Autodesk Fusion 360 part; units mm, degrees
(part 2 of 2)
  arc A318 (288.275, -92.225) -> (288.775, -92.725) centre (288.775, -92.225) ccw
  arc A319 (301.775, -92.725) -> (302.275, -92.225) centre (301.775, -92.225) ccw
  line L320 (5.4062, -97.775) -> (18.4063, -97.775)
  line L321 (5.4062, -111.775) -> (18.4063, -111.775)
  line L322 (4.9062, -98.275) -> (4.9062, -111.275)
  line L323 (18.9062, -98.275) -> (18.9062, -111.275)
  arc A320 (5.4062, -97.775) -> (4.9063, -98.275) centre (5.4062, -98.275) ccw
  arc A321 (18.9062, -98.275) -> (18.4062, -97.775) centre (18.4062, -98.275) ccw
  arc A322 (4.9062, -111.275) -> (5.4062, -111.775) centre (5.4062, -111.275) ccw
  arc A323 (18.4062, -111.775) -> (18.9063, -111.275) centre (18.4062, -111.275) ccw
  line L324 (29.2188, -97.775) -> (42.2188, -97.775)
  line L325 (29.2188, -111.775) -> (42.2188, -111.775)
  line L326 (28.7188, -98.275) -> (28.7188, -111.275)
  line L327 (42.7188, -98.275) -> (42.7188, -111.275)
  arc A324 (29.2188, -97.775) -> (28.7188, -98.275) centre (29.2188, -98.275) ccw
  arc A325 (42.7188, -98.275) -> (42.2188, -97.775) centre (42.2188, -98.275) ccw
  arc A326 (28.7188, -111.275) -> (29.2188, -111.775) centre (29.2188, -111.275) ccw
  arc A327 (42.2188, -111.775) -> (42.7188, -111.275) centre (42.2188, -111.275) ccw
  line L328 (53.0313, -97.775) -> (66.0312, -97.775)
  line L329 (53.0313, -111.775) -> (66.0312, -111.775)
  line L330 (52.5313, -98.275) -> (52.5313, -111.275)
  line L331 (66.5312, -98.275) -> (66.5312, -111.275)
  arc A328 (53.0313, -97.775) -> (52.5313, -98.275) centre (53.0313, -98.275) ccw
  arc A329 (66.5312, -98.275) -> (66.0312, -97.775) centre (66.0312, -98.275) ccw
  arc A330 (52.5313, -111.275) -> (53.0313, -111.775) centre (53.0313, -111.275) ccw
  arc A331 (66.0312, -111.775) -> (66.5312, -111.275) centre (66.0312, -111.275) ccw
  line L332 (124.4688, -97.775) -> (137.4688, -97.775)
  line L333 (124.4688, -111.775) -> (137.4688, -111.775)
  line L334 (123.9688, -98.275) -> (123.9688, -111.275)
  line L335 (137.9688, -98.275) -> (137.9688, -111.275)
  arc A332 (124.4688, -97.775) -> (123.9688, -98.275) centre (124.4688, -98.275) ccw
  arc A333 (137.9688, -98.275) -> (137.4688, -97.775) centre (137.4688, -98.275) ccw
  arc A334 (123.9688, -111.275) -> (124.4688, -111.775) centre (124.4688, -111.275) ccw
  arc A335 (137.4688, -111.775) -> (137.9688, -111.275) centre (137.4688, -111.275) ccw
  line L336 (77.9688, -98.775) -> (83.9688, -98.775)
  line L337 (77.9688, -113.775) -> (83.9688, -113.775)
  line L338 (77.4688, -99.275) -> (77.4688, -113.275)
  line L339 (84.4688, -99.275) -> (84.4688, -113.275)
  arc A336 (77.9688, -98.775) -> (77.4688, -99.275) centre (77.9688, -99.275) ccw
  arc A337 (84.4688, -99.275) -> (83.9688, -98.775) centre (83.9688, -99.275) ccw
  arc A338 (77.4688, -113.275) -> (77.9688, -113.775) centre (77.9688, -113.275) ccw
  arc A339 (83.9688, -113.775) -> (84.4688, -113.275) centre (83.9688, -113.275) ccw
  line L340 (177.9688, -98.775) -> (183.9688, -98.775)
  line L341 (177.9688, -113.775) -> (183.9688, -113.775)
  line L342 (177.4688, -99.275) -> (177.4688, -113.275)
  line L343 (184.4688, -99.275) -> (184.4688, -113.275)
  arc A340 (177.9688, -98.775) -> (177.4688, -99.275) centre (177.9688, -99.275) ccw
  arc A341 (184.4688, -99.275) -> (183.9688, -98.775) centre (183.9688, -99.275) ccw
  arc A342 (177.4688, -113.275) -> (177.9688, -113.775) centre (177.9688, -113.275) ccw
  arc A343 (183.9688, -113.775) -> (184.4688, -113.275) centre (183.9688, -113.275) ccw
  line L344 (193.525, -97.775) -> (206.525, -97.775)
  line L345 (193.525, -111.775) -> (206.525, -111.775)
  line L346 (193.025, -98.275) -> (193.025, -111.275)
  line L347 (207.025, -98.275) -> (207.025, -111.275)
  arc A344 (193.525, -97.775) -> (193.025, -98.275) centre (193.525, -98.275) ccw
  arc A345 (207.025, -98.275) -> (206.525, -97.775) centre (206.525, -98.275) ccw
  arc A346 (193.025, -111.275) -> (193.525, -111.775) centre (193.525, -111.275) ccw
  arc A347 (206.525, -111.775) -> (207.025, -111.275) centre (206.525, -111.275) ccw
  line L348 (212.575, -97.775) -> (225.575, -97.775)
  line L349 (212.575, -111.775) -> (225.575, -111.775)
  line L350 (212.075, -98.275) -> (212.075, -111.275)
  line L351 (226.075, -98.275) -> (226.075, -111.275)
  arc A348 (212.575, -97.775) -> (212.075, -98.275) centre (212.575, -98.275) ccw
  arc A349 (226.075, -98.275) -> (225.575, -97.775) centre (225.575, -98.275) ccw
  arc A350 (212.075, -111.275) -> (212.575, -111.775) centre (212.575, -111.275) ccw
  arc A351 (225.575, -111.775) -> (226.075, -111.275) centre (225.575, -111.275) ccw
  line L352 (231.625, -97.775) -> (244.625, -97.775)
  line L353 (231.625, -111.775) -> (244.625, -111.775)
  line L354 (231.125, -98.275) -> (231.125, -111.275)
  line L355 (245.125, -98.275) -> (245.125, -111.275)
  arc A352 (231.625, -97.775) -> (231.125, -98.275) centre (231.625, -98.275) ccw
  arc A353 (245.125, -98.275) -> (244.625, -97.775) centre (244.625, -98.275) ccw
  arc A354 (231.125, -111.275) -> (231.625, -111.775) centre (231.625, -111.275) ccw
  arc A355 (244.625, -111.775) -> (245.125, -111.275) centre (244.625, -111.275) ccw
  line L356 (250.675, -97.775) -> (263.675, -97.775)
  line L357 (250.675, -111.775) -> (263.675, -111.775)
  line L358 (250.175, -98.275) -> (250.175, -111.275)
  line L359 (264.175, -98.275) -> (264.175, -111.275)
  arc A356 (250.675, -97.775) -> (250.175, -98.275) centre (250.675, -98.275) ccw
  arc A357 (264.175, -98.275) -> (263.675, -97.775) centre (263.675, -98.275) ccw
  arc A358 (250.175, -111.275) -> (250.675, -111.775) centre (250.675, -111.275) ccw
  arc A359 (263.675, -111.775) -> (264.175, -111.275) centre (263.675, -111.275) ccw
  line L360 (269.725, -97.775) -> (282.725, -97.775)
  line L361 (269.725, -111.775) -> (282.725, -111.775)
  line L362 (269.225, -98.275) -> (269.225, -111.275)
  line L363 (283.225, -98.275) -> (283.225, -111.275)
  arc A360 (269.725, -97.775) -> (269.225, -98.275) centre (269.725, -98.275) ccw
  arc A361 (283.225, -98.275) -> (282.725, -97.775) centre (282.725, -98.275) ccw
  arc A362 (269.225, -111.275) -> (269.725, -111.775) centre (269.725, -111.275) ccw
  arc A363 (282.725, -111.775) -> (283.225, -111.275) centre (282.725, -111.275) ccw
  line L364 (288.775, -97.775) -> (301.775, -97.775)
  line L365 (288.775, -111.775) -> (301.775, -111.775)
  line L366 (288.275, -98.275) -> (288.275, -111.275)
  line L367 (302.275, -98.275) -> (302.275, -111.275)
  arc A364 (288.775, -97.775) -> (288.275, -98.275) centre (288.775, -98.275) ccw
  arc A365 (302.275, -98.275) -> (301.775, -97.775) centre (301.775, -98.275) ccw
  arc A366 (288.275, -111.275) -> (288.775, -111.775) centre (288.775, -111.275) ccw
  arc A367 (301.775, -111.775) -> (302.275, -111.275) centre (301.775, -111.275) ccw
sketch "Sketch2" plane through (0, 0, 0) normal (0, 0, 1) x (1, 0, 0)
  line L0 (-12.5938, 18.225) -> (358.4062, 18.225)
  line L1 (358.4062, 18.225) -> (358.4062, -133.775)
  line L2 (358.4062, -133.775) -> (-12.5938, -133.775)
  line L3 (-12.5938, -133.775) -> (-12.5938, 18.225)
  line L4 (5.4062, -111.775) -> (18.4063, -111.775)
  line L5 (4.9062, -98.275) -> (4.9062, -111.275)
  dimension "d1" = 371
  dimension "d2" = 152
  dimension "d3" = 22
  dimension "d4" = 17.5
  constraint horizontal L0
  constraint vertical L1
  constraint horizontal L2
  constraint vertical L3
  measures "d1" distance of L0.start L0.end
  measures "d2" distance of L0.start L2.end
  measures "d3" distance of L2 L4
  measures "d4" distance of L3 L5
sketch "Sketch3" plane through (0, 0, 0) normal (0, 0, 1) x (1, 0, 0)
  circle A0 centre (353.4062, 13.225) radius 1.7
  line L0 (-12.5938, 18.225) -> (358.4062, 18.225)
  line L1 (358.4062, 18.225) -> (358.4062, -133.775)
  circle A1 centre (-7.5937, 13.225) radius 1.7
  line L2 (-12.5938, -133.775) -> (-12.5938, 18.225)
  circle A2 centre (-7.5938, -128.775) radius 1.7
  line L3 (358.4062, -133.775) -> (-12.5938, -133.775)
  circle A3 centre (353.4062, -128.775) radius 1.7
  circle A4 centre (-7.5938, 13.225) radius 3
  circle A5 centre (353.4062, 13.225) radius 3
  circle A6 centre (353.4062, -128.775) radius 3
  circle A7 centre (-7.5937, -128.775) radius 3
  dimension "d5" = 3.4
  dimension "d6" = 5
  dimension "d7" = 5
  dimension "d8" = 3.4
  dimension "d9" = 5
  dimension "d10" = 5
  dimension "d11" = 3.4
  dimension "d12" = 5
  dimension "d13" = 5
  dimension "d14" = 3.4
  dimension "d15" = 5
  dimension "d16" = 5
  dimension "d17" = 6
  dimension "d18" = 6
  dimension "d19" = 6
  dimension "d20" = 6
  constraint coincident A1.centre A4.centre
  constraint coincident A2.centre A7.centre
  constraint coincident A3.centre A6.centre
  constraint coincident A0.centre A5.centre
  measures "d5" diameter of A0
  measures "d6" distance of A0.centre L0
  measures "d7" distance of A0.centre L1
  measures "d8" diameter of A1
  measures "d9" distance of A1.centre L2
  measures "d10" distance of L0 A1.centre
  measures "d11" diameter of A2
  measures "d12" distance of A2.centre L3
  measures "d13" distance of L2 A2.centre
  measures "d14" diameter of A3
  measures "d15" distance of L3 A3.centre
  measures "d16" distance of L1 A3.centre
  measures "d17" diameter of A4
  measures "d18" diameter of A5
  measures "d19" diameter of A6
  measures "d20" diameter of A7
extrude "Extrude1" add sketch "Sketch3" along normal blind 1.5 contours L0 L1 L2 L3
extrude "Extrude2" cut sketch "plate-2026-01-22T00_34_46.063Z" along normal blind 1.5
